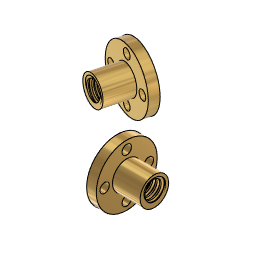
T8 Screw nut (Autodesk Fusion 360 design; units mm, degrees)
Autodesk Fusion 360 part; units mm, degrees
sketch "Sketch1" plane through (0, 0, 0) normal (1, 0, 0) x (0, 1, 0)
  circle A0 centre (0, 0) radius 11
  circle A1 centre (0, 0) radius 5.15
  circle A2 centre (0, 0) radius 3.5
  line L0 (11, 0) -> (-11, 0) construction
  line L1 (0, -11) -> (0, 11) construction
  circle A3 centre (0, 8) radius 1.7
  line L2 (0, 11) -> (0, 8)
  circle A4 centre (-8, 0) radius 1.7
  circle A5 centre (0, -8) radius 1.7
  circle A6 centre (8, 0) radius 1.7
  dimension "d1" = 22
  dimension "d2" = 10.3
  dimension "d7" = 7
  dimension "d10" = 3.4
  dimension "d11" = 3
  dimension "d13" = 360
  constraint coincident A0.centre A1.centre
  constraint coincident A0 L1.end
  constraint coincident A0 L0.start
  constraint coincident A0 L0.end
  constraint coincident A0 L1.start
  constraint perpendicular L0 L1
  constraint coincident L1 A3.centre
  constraint coincident A3.centre L2.end
  measures "d1" diameter of A0
  measures "d2" diameter of A1
  measures "d7" diameter of A2
  measures "d10" diameter of A3
  measures "d11" distance of L1.end A3.centre
extrude "Extrude1" add sketch "Sketch1" along normal blind 3.5 contours A0 | A3 | A4 | A5 | A6 makes body 1
move_body "Move1" bodies 1 to x (1, 0, 0) y (0, 1, 0) z (0, 0, 1) at (1.5, 0, 0)
extrude "Extrude2" add sketch "Sketch1" along normal blind 15 contours A1 | A2 bodies 1
extrude "Extrude3" cut sketch "Sketch1" along normal blind 23 contours A2 bodies 1
thread "Thread1" "ISO Metric Trapezoidal Threads 8.0 TR8x1.5 7H" major diameter 8.3 minor diameter 6.595 pitch 1.5 angle 30 modelled right hand crest width 0.5445 on face at (10, 3.4826, 0.3485) crest through (0.375, 3.2975, 0) on bodies 1
extrude "Extrude4" cut sketch "Sketch1" along normal blind 8 contours A3 | A4 | A5 | A6 bodies 1
copy_body "CopyPasteBodies1" bodies 1 makes body 2
move_body "Move5" bodies 2 to x (1, 0, 0) y (0, 1, 0) z (0, 0, 1) at (0, 0, 30)
move_body "Move6" bodies 2 to x (-0.258819, -0.965926, 0) y (0.965926, -0.258819, 0) z (0, 0, 1) at (6.2941, 4.8296, 0)
move_body "Move2" [rolled back]
ref_plane "WorkPlane1" through (18, 0, 0) normal (1, 0, 0) x (0, 1, 0)
sketch "Sketch4" plane through (18, 0, 0) normal (1, 0, 0) x (0, 1, 0)
  circle A0 centre (0, 8) radius 3.5
  circle A1 centre (0, 8) radius 1.75
  circle A2 centre (0, 8) radius 2.75
  circle A3 centre (0, 8) radius 1.5
  dimension "d17" = 7
  dimension "d18" = 3.5
  dimension "d19" = 5.5
  dimension "d20" = 3
  constraint concentric A0 A1
  constraint concentric A1 A2
  constraint concentric A1 A3
  measures "d17" diameter of A0
  measures "d18" diameter of A1
  measures "d19" diameter of A2
  measures "d20" diameter of A3
extrude "Extrude5" [rolled back] along distance 3 taper angle 0
move_body "Move3" [rolled back]
extrude "Extrude6" [rolled back] along distance 0.6 taper angle 0
extrude "Extrude7" [rolled back] along distance 0.9 taper angle 0
extrude "Extrude8" [rolled back] along distance -34.5 taper angle 0
thread "Thread2" [rolled back]
chamfer "Chamfer1" [rolled back] distance 0.1
chamfer "Chamfer2" [rolled back] distance 0.1
sketch "Sketch5" plane through (21.6, 0, 0) normal (1, 0, 0) x (0, 1, 0)
  circle A0 centre (0, 8) radius 2.65
  line L0 (-0.7217, 9.25) -> (-1.4434, 8)
  line L1 (-1.4434, 8) -> (-0.7217, 6.75)
  line L2 (-0.7217, 6.75) -> (0.7217, 6.75)
  line L3 (0.7217, 6.75) -> (1.4434, 8)
  line L4 (1.4434, 8) -> (0.7217, 9.25)
  line L5 (0.7217, 9.25) -> (-0.7217, 9.25)
  point P0 (0, 8)
  dimension "d31" = 1.25
  constraint coincident P0 A0.centre
  measures "d31" distance of P0 L5
extrude "Extrude9" [rolled back] along distance -2 taper angle 0
coilprimitive "CoilPrimitive1" [rolled back] diameter 5 section size 0.5 taper angle 0 height -13
move_body "Move4" [rolled back]
sketch "Sketch7" plane through (-13.5, 0, 0) normal (-1, 0, 0) x (0, -1, 0)
  circle A0 centre (8, 0) radius 1.7
  circle A1 centre (0, -8) radius 1.7
  circle A2 centre (0, 8) radius 1.7
  circle A3 centre (-8, 0) radius 1.7
  circle A4 centre (0, 0) radius 5.15
  circle A5 centre (0, 0) radius 11
  line L0 (-1.5877, 10.75) -> (-3.1754, 8)
  line L1 (-3.1754, 8) -> (-1.5877, 5.25)
  line L2 (-1.5877, 5.25) -> (1.5877, 5.25)
  line L3 (1.5877, 5.25) -> (3.1754, 8)
  line L4 (3.1754, 8) -> (1.5877, 10.75)
  line L5 (1.5877, 10.75) -> (-1.5877, 10.75)
  point P0 (0, 8)
  dimension "d39" = 2.75
  constraint coincident P0 A2.centre
  measures "d39" distance of P0 L5
extrude "Extrude10" [rolled back] along distance 2.5 taper angle 0
thread "Thread3" [rolled back]
ref_plane "WorkPlane4" through (-14.75, 0, 8) normal (0, 0, -1) x (0, -1, 0)
sketch "Sketch9" plane through (-14.75, 0, 8) normal (0, 0, -1) x (1, 0, 0)
  line L0 (-1.0442, -3.1797) -> (-1.3, -3.4)
  line L1 (-1.3, -3.4) -> (-1.25, 0)
  line L2 (0, 0) -> (0, -3.2)
  line L3 (1.0442, -3.1797) -> (1.3, -3.4)
  line L4 (1.3, -3.4) -> (1.25, 0)
  line L5 (-1.25, 0) -> (1.25, 0)
  arc A0 (-1.2711, -1.4381) -> (-1.0442, -3.1797) centre (4.8363, -1.5279) ccw
  arc A1 (1.0442, -3.1797) -> (1.2711, -1.4381) centre (-4.8363, -1.5279) ccw
  constraint coincident L2.start origin
  constraint vertical L2
  constraint symmetric L1.end L2 L4.end
  constraint symmetric L0.start L2 L3.start
  constraint symmetric L0.end L2 L3.end
  constraint tangent L1 A0
  constraint coincident L1 A0.start
  constraint symmetric L2 A0.start A1.end
  constraint symmetric L2 A0 A1
revolve "Revolve1" [rolled back] along angle 360
pattern_circular "C-Pattern1" [rolled back] total angle 360
equation "d31 = ( 2.5 / 2 ) * 1 mm"
equation "d39 = ( 5.5 / 2 ) * 1 mm"
